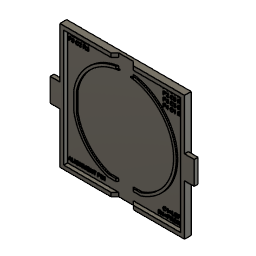
pin_grid_wafer_jig (Autodesk Fusion 360 design; units mm, degrees)
part number: 2026-08-11-19-59-54-396
Autodesk Fusion 360 part; units mm, degrees
ref_plane "WorkPlane1" through (0, 0, 3) normal (0, 0, 1) x (1, 0, 0)
ref_plane "WorkPlane2" through (0, 0, 4.7) normal (0, 0, 1) x (1, 0, 0)
ref_plane "WorkPlane3" through (0, 0, 7.2) normal (0, 0, 1) x (1, 0, 0)
ref_plane "WorkPlane4" through (0, 0, -5) normal (0, 0, 1) x (1, 0, 0)
ref_plane "WorkPlane5" through (0, 0, -4) normal (0, 0, 1) x (1, 0, 0)
sketch "128 mm Square Wafer Platform Sketch" plane through (0, 0, 0) normal (0, 0, 1) x (1, 0, 0)
  line L0 (-53.693, -70.236) -> (74.307, -70.236)
  line L1 (74.307, -70.236) -> (74.307, 57.764)
  line L2 (74.307, 57.764) -> (-53.693, 57.764)
  line L3 (-53.693, 57.764) -> (-53.693, -70.236)
extrude "128 mm Square Wafer Platform" add sketch "128 mm Square Wafer Platform Sketch" along normal blind 3
sketch "4 x 4 mm Perimeter Reinforcement Bar Sketch" plane through (0, 0, 3) normal (0, 0, 1) x (1, 0, 0)
  line L0 (-53.693, -70.236) -> (74.307, -70.236)
  line L1 (74.307, -70.236) -> (74.307, 57.764)
  line L2 (74.307, 57.764) -> (-53.693, 57.764)
  line L3 (-53.693, 57.764) -> (-53.693, -70.236)
  line L4 (-49.693, -66.236) -> (70.307, -66.236)
  line L5 (70.307, -66.236) -> (70.307, 53.764)
  line L6 (70.307, 53.764) -> (-49.693, 53.764)
  line L7 (-49.693, 53.764) -> (-49.693, -66.236)
extrude "4 x 4 mm Perimeter Reinforcement Bar" add sketch "4 x 4 mm Perimeter Reinforcement Bar Sketch" along normal blind 4
sketch "Left Pickup Tab Sketch" plane through (0, 0, 3) normal (0, 0, 1) x (1, 0, 0)
  line L0 (-63.693, -18.236) -> (-53.693, -18.236)
  line L1 (-53.693, -18.236) -> (-53.693, 5.764)
  line L2 (-53.693, 5.764) -> (-63.693, 5.764)
  line L3 (-63.693, 5.764) -> (-63.693, -18.236)
extrude "Left Pickup Tab" add sketch "Left Pickup Tab Sketch" along normal blind 4
sketch "Right Pickup Tab Sketch" plane through (0, 0, 3) normal (0, 0, 1) x (1, 0, 0)
  line L0 (74.307, -18.236) -> (84.307, -18.236)
  line L1 (84.307, -18.236) -> (84.307, 5.764)
  line L2 (84.307, 5.764) -> (74.307, 5.764)
  line L3 (74.307, 5.764) -> (74.307, -18.236)
extrude "Right Pickup Tab" add sketch "Right Pickup Tab Sketch" along normal blind 4
sketch "15 mm Outer Bar Tweezer Notch with 45 Degree Sides Lower Sketch" plane through (0, 0, 3) normal (0, 0, 1) x (1, 0, 0)
  line L0 (2.807, -70.336) -> (17.807, -70.336)
  line L1 (17.807, -70.336) -> (17.807, -66.136)
  line L2 (17.807, -66.136) -> (2.807, -66.136)
  line L3 (2.807, -66.136) -> (2.807, -70.336)
sketch "15 mm Outer Bar Tweezer Notch with 45 Degree Sides Upper Sketch" plane through (0, 0, 7.2) normal (0, 0, 1) x (1, 0, 0)
  line L0 (-1.393, -74.536) -> (22.007, -74.536)
  line L1 (22.007, -74.536) -> (22.007, -61.936)
  line L2 (22.007, -61.936) -> (-1.393, -61.936)
  line L3 (-1.393, -61.936) -> (-1.393, -74.536)
loft "15 mm Outer Bar Tweezer Notch with 45 Degree Sides" cut profiles "15 mm Outer Bar Tweezer Notch with 45 Degree Sides Lower Sketch", "15 mm Outer Bar Tweezer Notch with 45 Degree Sides Upper Sketch" section 1 section 2
sketch "1.5 mm Raised Wafer Nest Sketch" plane through (0, 0, 3) normal (0, 0, 1) x (1, 0, 0)
  line L0 (63.307, -6.236) -> (63.2747, -4.3863)
  line L1 (63.2747, -4.3863) -> (63.1779, -2.5389)
  line L2 (63.1779, -2.5389) -> (63.0167, -0.696)
  line L3 (63.0167, -0.696) -> (62.7912, 1.1402)
  line L4 (62.7912, 1.1402) -> (62.5018, 2.9674)
  line L5 (62.5018, 2.9674) -> (62.1488, 4.7833)
  line L6 (62.1488, 4.7833) -> (61.7327, 6.5859)
  line L7 (61.7327, 6.5859) -> (61.2539, 8.3728)
  line L8 (61.2539, 8.3728) -> (60.713, 10.1419)
  line L9 (60.713, 10.1419) -> (60.1107, 11.8911)
  line L10 (60.1107, 11.8911) -> (59.4477, 13.6181)
  line L11 (59.4477, 13.6181) -> (58.7249, 15.321)
  line L12 (58.7249, 15.321) -> (57.9431, 16.9977)
  line L13 (57.9431, 16.9977) -> (57.1032, 18.646)
  line L14 (57.1032, 18.646) -> (56.2063, 20.264)
  line L15 (56.2063, 20.264) -> (55.2535, 21.8497)
  line L16 (55.2535, 21.8497) -> (54.246, 23.4012)
  line L17 (54.246, 23.4012) -> (53.1849, 24.9166)
  line L18 (53.1849, 24.9166) -> (52.0716, 26.3941)
  line L19 (52.0716, 26.3941) -> (50.9074, 27.8317)
  line L20 (50.9074, 27.8317) -> (49.6937, 29.2279)
  line L21 (49.6937, 29.2279) -> (48.432, 30.5809)
  line L22 (48.432, 30.5809) -> (47.1239, 31.889)
  line L23 (47.1239, 31.889) -> (45.7709, 33.1507)
  line L24 (45.7709, 33.1507) -> (44.3747, 34.3644)
  line L25 (44.3747, 34.3644) -> (42.9371, 35.5286)
  line L26 (42.9371, 35.5286) -> (41.4596, 36.6419)
  line L27 (41.4596, 36.6419) -> (39.9442, 37.703)
  line L28 (39.9442, 37.703) -> (38.3927, 38.7105)
  line L29 (38.3927, 38.7105) -> (36.807, 39.6633)
  line L30 (36.807, 39.6633) -> (35.189, 40.5602)
  line L31 (35.189, 40.5602) -> (33.5407, 41.4001)
  line L32 (33.5407, 41.4001) -> (31.864, 42.1819)
  line L33 (31.864, 42.1819) -> (30.1611, 42.9047)
  line L34 (30.1611, 42.9047) -> (28.4341, 43.5677)
  line L35 (28.4341, 43.5677) -> (26.6849, 44.17)
  line L36 (26.6849, 44.17) -> (24.9158, 44.7109)
  line L37 (24.9158, 44.7109) -> (23.1289, 45.1897)
  line L38 (23.1289, 45.1897) -> (21.3263, 45.6058)
  line L39 (21.3263, 45.6058) -> (19.5104, 45.9588)
  line L40 (19.5104, 45.9588) -> (17.6832, 46.2482)
  line L41 (17.6832, 46.2482) -> (15.847, 46.4737)
  line L42 (15.847, 46.4737) -> (14.0041, 46.6349)
  line L43 (14.0041, 46.6349) -> (12.1567, 46.7317)
  line L44 (12.1567, 46.7317) -> (10.307, 46.764)
  line L45 (10.307, 46.764) -> (8.4573, 46.7317)
  line L46 (8.4573, 46.7317) -> (6.6099, 46.6349)
  line L47 (6.6099, 46.6349) -> (4.767, 46.4737)
  line L48 (4.767, 46.4737) -> (2.9308, 46.2482)
  line L49 (2.9308, 46.2482) -> (1.1036, 45.9588)
  line L50 (1.1036, 45.9588) -> (-0.7123, 45.6058)
  line L51 (-0.7123, 45.6058) -> (-2.5149, 45.1897)
  line L52 (-2.5149, 45.1897) -> (-4.3018, 44.7109)
  line L53 (-4.3018, 44.7109) -> (-6.0709, 44.17)
  line L54 (-6.0709, 44.17) -> (-7.8201, 43.5677)
  line L55 (-7.8201, 43.5677) -> (-9.5471, 42.9047)
  line L56 (-9.5471, 42.9047) -> (-11.25, 42.1819)
  line L57 (-11.25, 42.1819) -> (-12.9267, 41.4001)
  line L58 (-12.9267, 41.4001) -> (-14.575, 40.5602)
  line L59 (-14.575, 40.5602) -> (-16.193, 39.6633)
  line L60 (-16.193, 39.6633) -> (-17.7787, 38.7105)
  line L61 (-17.7787, 38.7105) -> (-19.3302, 37.703)
  line L62 (-19.3302, 37.703) -> (-20.8456, 36.6419)
  line L63 (-20.8456, 36.6419) -> (-22.3231, 35.5286)
  line L64 (-22.3231, 35.5286) -> (-23.7607, 34.3644)
  line L65 (-23.7607, 34.3644) -> (-25.1569, 33.1507)
  line L66 (-25.1569, 33.1507) -> (-26.5099, 31.889)
  line L67 (-26.5099, 31.889) -> (-27.818, 30.5809)
  line L68 (-27.818, 30.5809) -> (-29.0797, 29.2279)
  line L69 (-29.0797, 29.2279) -> (-30.2934, 27.8317)
  line L70 (-30.2934, 27.8317) -> (-31.4576, 26.3941)
  line L71 (-31.4576, 26.3941) -> (-32.5709, 24.9166)
  line L72 (-32.5709, 24.9166) -> (-33.632, 23.4012)
  line L73 (-33.632, 23.4012) -> (-34.6395, 21.8497)
  line L74 (-34.6395, 21.8497) -> (-35.5923, 20.264)
  line L75 (-35.5923, 20.264) -> (-36.4892, 18.646)
  line L76 (-36.4892, 18.646) -> (-37.3291, 16.9977)
  line L77 (-37.3291, 16.9977) -> (-38.1109, 15.321)
  line L78 (-38.1109, 15.321) -> (-38.8337, 13.6181)
  line L79 (-38.8337, 13.6181) -> (-39.4967, 11.8911)
  line L80 (-39.4967, 11.8911) -> (-40.099, 10.1419)
  line L81 (-40.099, 10.1419) -> (-40.6399, 8.3728)
  line L82 (-40.6399, 8.3728) -> (-41.1187, 6.5859)
  line L83 (-41.1187, 6.5859) -> (-41.5348, 4.7833)
  line L84 (-41.5348, 4.7833) -> (-41.8763, 3.0264)
  line L85 (-41.8763, 3.0264) -> (-41.8763, -15.4984)
  line L86 (-41.8763, -15.4984) -> (-41.5348, -17.2553)
  line L87 (-41.5348, -17.2553) -> (-41.1187, -19.0579)
  line L88 (-41.1187, -19.0579) -> (-40.6399, -20.8448)
  line L89 (-40.6399, -20.8448) -> (-40.099, -22.6139)
  line L90 (-40.099, -22.6139) -> (-39.4967, -24.3631)
  line L91 (-39.4967, -24.3631) -> (-38.8337, -26.0901)
  line L92 (-38.8337, -26.0901) -> (-38.1109, -27.793)
  line L93 (-38.1109, -27.793) -> (-37.3291, -29.4697)
  line L94 (-37.3291, -29.4697) -> (-36.4892, -31.118)
  line L95 (-36.4892, -31.118) -> (-35.5923, -32.736)
  line L96 (-35.5923, -32.736) -> (-34.6395, -34.3217)
  line L97 (-34.6395, -34.3217) -> (-33.632, -35.8732)
  line L98 (-33.632, -35.8732) -> (-32.5709, -37.3886)
  line L99 (-32.5709, -37.3886) -> (-31.4576, -38.8661)
  line L100 (-31.4576, -38.8661) -> (-30.2934, -40.3037)
  line L101 (-30.2934, -40.3037) -> (-29.0797, -41.6999)
  line L102 (-29.0797, -41.6999) -> (-27.818, -43.0529)
  line L103 (-27.818, -43.0529) -> (-26.5099, -44.361)
  line L104 (-26.5099, -44.361) -> (-25.1569, -45.6227)
  line L105 (-25.1569, -45.6227) -> (-23.7607, -46.8364)
  line L106 (-23.7607, -46.8364) -> (-22.3231, -48.0006)
  line L107 (-22.3231, -48.0006) -> (-20.8456, -49.1139)
  line L108 (-20.8456, -49.1139) -> (-19.3302, -50.175)
  line L109 (-19.3302, -50.175) -> (-17.7787, -51.1825)
  line L110 (-17.7787, -51.1825) -> (-16.193, -52.1353)
  line L111 (-16.193, -52.1353) -> (-14.575, -53.0322)
  line L112 (-14.575, -53.0322) -> (-12.9267, -53.8721)
  line L113 (-12.9267, -53.8721) -> (-11.25, -54.6539)
  line L114 (-11.25, -54.6539) -> (-9.5471, -55.3767)
  line L115 (-9.5471, -55.3767) -> (-7.8201, -56.0397)
  line L116 (-7.8201, -56.0397) -> (-6.4203, -56.5217)
  line L117 (-6.4203, -56.5217) -> (27.0343, -56.5217)
  line L118 (27.0343, -56.5217) -> (28.4341, -56.0397)
  line L119 (28.4341, -56.0397) -> (30.1611, -55.3767)
  line L120 (30.1611, -55.3767) -> (31.864, -54.6539)
  line L121 (31.864, -54.6539) -> (33.5407, -53.8721)
  line L122 (33.5407, -53.8721) -> (35.189, -53.0322)
  line L123 (35.189, -53.0322) -> (36.807, -52.1353)
  line L124 (36.807, -52.1353) -> (38.3927, -51.1825)
  line L125 (38.3927, -51.1825) -> (39.9442, -50.175)
  line L126 (39.9442, -50.175) -> (41.4596, -49.1139)
  line L127 (41.4596, -49.1139) -> (42.9371, -48.0006)
  line L128 (42.9371, -48.0006) -> (44.3747, -46.8364)
  line L129 (44.3747, -46.8364) -> (45.7709, -45.6227)
  line L130 (45.7709, -45.6227) -> (47.1239, -44.361)
  line L131 (47.1239, -44.361) -> (48.432, -43.0529)
  line L132 (48.432, -43.0529) -> (49.6937, -41.6999)
  line L133 (49.6937, -41.6999) -> (50.9074, -40.3037)
  line L134 (50.9074, -40.3037) -> (52.0716, -38.8661)
  line L135 (52.0716, -38.8661) -> (53.1849, -37.3886)
  line L136 (53.1849, -37.3886) -> (54.246, -35.8732)
  line L137 (54.246, -35.8732) -> (55.2535, -34.3217)
  line L138 (55.2535, -34.3217) -> (56.2063, -32.736)
  line L139 (56.2063, -32.736) -> (57.1032, -31.118)
  line L140 (57.1032, -31.118) -> (57.9431, -29.4697)
  line L141 (57.9431, -29.4697) -> (58.7249, -27.793)
  line L142 (58.7249, -27.793) -> (59.4477, -26.0901)
  line L143 (59.4477, -26.0901) -> (60.1107, -24.3631)
  line L144 (60.1107, -24.3631) -> (60.713, -22.6139)
  line L145 (60.713, -22.6139) -> (61.2539, -20.8448)
  line L146 (61.2539, -20.8448) -> (61.7327, -19.0579)
  line L147 (61.7327, -19.0579) -> (62.1488, -17.2553)
  line L148 (62.1488, -17.2553) -> (62.5018, -15.4394)
  line L149 (62.5018, -15.4394) -> (62.7912, -13.6122)
  line L150 (62.7912, -13.6122) -> (63.0167, -11.776)
  line L151 (63.0167, -11.776) -> (63.1779, -9.9331)
  line L152 (63.1779, -9.9331) -> (63.2747, -8.0857)
  line L153 (63.2747, -8.0857) -> (63.307, -6.236)
extrude "1.5 mm Raised Wafer Nest" add sketch "1.5 mm Raised Wafer Nest Sketch" along normal blind 1.5
sketch "Final Wafer Pocket Clearance Sketch" plane through (0, 0, 3) normal (0, 0, 1) x (1, 0, 0)
  line L0 (60.632, -6.236) -> (60.6013, -4.4797)
  line L1 (60.6013, -4.4797) -> (60.5094, -2.7255)
  line L2 (60.5094, -2.7255) -> (60.3563, -0.9756)
  line L3 (60.3563, -0.9756) -> (60.1422, 0.7679)
  line L4 (60.1422, 0.7679) -> (59.8675, 2.5028)
  line L5 (59.8675, 2.5028) -> (59.5323, 4.2272)
  line L6 (59.5323, 4.2272) -> (59.1371, 5.9387)
  line L7 (59.1371, 5.9387) -> (58.6825, 7.6354)
  line L8 (58.6825, 7.6354) -> (58.1689, 9.3153)
  line L9 (58.1689, 9.3153) -> (57.597, 10.9762)
  line L10 (57.597, 10.9762) -> (56.9675, 12.6161)
  line L11 (56.9675, 12.6161) -> (56.2812, 14.233)
  line L12 (56.2812, 14.233) -> (55.5388, 15.825)
  line L13 (55.5388, 15.825) -> (54.7413, 17.3902)
  line L14 (54.7413, 17.3902) -> (53.8897, 18.9265)
  line L15 (53.8897, 18.9265) -> (52.985, 20.4322)
  line L16 (52.985, 20.4322) -> (52.0283, 21.9054)
  line L17 (52.0283, 21.9054) -> (51.0208, 23.3443)
  line L18 (51.0208, 23.3443) -> (49.9636, 24.7472)
  line L19 (49.9636, 24.7472) -> (48.8582, 26.1123)
  line L20 (48.8582, 26.1123) -> (47.7058, 27.438)
  line L21 (47.7058, 27.438) -> (46.5078, 28.7227)
  line L22 (46.5078, 28.7227) -> (45.2657, 29.9648)
  line L23 (45.2657, 29.9648) -> (43.981, 31.1628)
  line L24 (43.981, 31.1628) -> (42.6553, 32.3152)
  line L25 (42.6553, 32.3152) -> (41.2902, 33.4206)
  line L26 (41.2902, 33.4206) -> (39.8873, 34.4778)
  line L27 (39.8873, 34.4778) -> (38.4484, 35.4853)
  line L28 (38.4484, 35.4853) -> (36.9752, 36.442)
  line L29 (36.9752, 36.442) -> (35.4695, 37.3467)
  line L30 (35.4695, 37.3467) -> (33.9332, 38.1983)
  line L31 (33.9332, 38.1983) -> (32.368, 38.9958)
  line L32 (32.368, 38.9958) -> (30.776, 39.7382)
  line L33 (30.776, 39.7382) -> (29.1591, 40.4245)
  line L34 (29.1591, 40.4245) -> (27.5192, 41.054)
  line L35 (27.5192, 41.054) -> (25.8583, 41.6259)
  line L36 (25.8583, 41.6259) -> (24.1784, 42.1395)
  line L37 (24.1784, 42.1395) -> (22.4817, 42.5941)
  line L38 (22.4817, 42.5941) -> (20.7702, 42.9893)
  line L39 (20.7702, 42.9893) -> (19.0458, 43.3245)
  line L40 (19.0458, 43.3245) -> (17.3109, 43.5992)
  line L41 (17.3109, 43.5992) -> (15.5674, 43.8133)
  line L42 (15.5674, 43.8133) -> (13.8175, 43.9664)
  line L43 (13.8175, 43.9664) -> (12.0633, 44.0583)
  line L44 (12.0633, 44.0583) -> (10.307, 44.089)
  line L45 (10.307, 44.089) -> (8.5507, 44.0583)
  line L46 (8.5507, 44.0583) -> (6.7965, 43.9664)
  line L47 (6.7965, 43.9664) -> (5.0466, 43.8133)
  line L48 (5.0466, 43.8133) -> (3.3031, 43.5992)
  line L49 (3.3031, 43.5992) -> (1.5682, 43.3245)
  line L50 (1.5682, 43.3245) -> (-0.1562, 42.9893)
  line L51 (-0.1562, 42.9893) -> (-1.8677, 42.5941)
  line L52 (-1.8677, 42.5941) -> (-3.5644, 42.1395)
  line L53 (-3.5644, 42.1395) -> (-5.2443, 41.6259)
  line L54 (-5.2443, 41.6259) -> (-6.9052, 41.054)
  line L55 (-6.9052, 41.054) -> (-8.5451, 40.4245)
  line L56 (-8.5451, 40.4245) -> (-10.162, 39.7382)
  line L57 (-10.162, 39.7382) -> (-11.754, 38.9958)
  line L58 (-11.754, 38.9958) -> (-13.3192, 38.1983)
  line L59 (-13.3192, 38.1983) -> (-14.8555, 37.3467)
  line L60 (-14.8555, 37.3467) -> (-16.3612, 36.442)
  line L61 (-16.3612, 36.442) -> (-17.8344, 35.4853)
  line L62 (-17.8344, 35.4853) -> (-19.2733, 34.4778)
  line L63 (-19.2733, 34.4778) -> (-20.6762, 33.4206)
  line L64 (-20.6762, 33.4206) -> (-22.0413, 32.3152)
  line L65 (-22.0413, 32.3152) -> (-23.367, 31.1628)
  line L66 (-23.367, 31.1628) -> (-24.6517, 29.9648)
  line L67 (-24.6517, 29.9648) -> (-25.8938, 28.7227)
  line L68 (-25.8938, 28.7227) -> (-27.0918, 27.438)
  line L69 (-27.0918, 27.438) -> (-28.2442, 26.1123)
  line L70 (-28.2442, 26.1123) -> (-29.3496, 24.7472)
  line L71 (-29.3496, 24.7472) -> (-30.4068, 23.3443)
  line L72 (-30.4068, 23.3443) -> (-31.4143, 21.9054)
  line L73 (-31.4143, 21.9054) -> (-32.371, 20.4322)
  line L74 (-32.371, 20.4322) -> (-33.2757, 18.9265)
  line L75 (-33.2757, 18.9265) -> (-34.1273, 17.3902)
  line L76 (-34.1273, 17.3902) -> (-34.9248, 15.825)
  line L77 (-34.9248, 15.825) -> (-35.6672, 14.233)
  line L78 (-35.6672, 14.233) -> (-36.3535, 12.6161)
  line L79 (-36.3535, 12.6161) -> (-36.983, 10.9762)
  line L80 (-36.983, 10.9762) -> (-37.5549, 9.3153)
  line L81 (-37.5549, 9.3153) -> (-38.0685, 7.6354)
  line L82 (-38.0685, 7.6354) -> (-38.5231, 5.9387)
  line L83 (-38.5231, 5.9387) -> (-38.9183, 4.2272)
  line L84 (-38.9183, 4.2272) -> (-39.0713, 3.4398)
  line L85 (-39.0713, 3.4398) -> (-39.0713, -15.9118)
  line L86 (-39.0713, -15.9118) -> (-38.9183, -16.6992)
  line L87 (-38.9183, -16.6992) -> (-38.5231, -18.4107)
  line L88 (-38.5231, -18.4107) -> (-38.0685, -20.1074)
  line L89 (-38.0685, -20.1074) -> (-37.5549, -21.7873)
  line L90 (-37.5549, -21.7873) -> (-36.983, -23.4482)
  line L91 (-36.983, -23.4482) -> (-36.3535, -25.0881)
  line L92 (-36.3535, -25.0881) -> (-35.6672, -26.705)
  line L93 (-35.6672, -26.705) -> (-34.9248, -28.297)
  line L94 (-34.9248, -28.297) -> (-34.1273, -29.8622)
  line L95 (-34.1273, -29.8622) -> (-33.2757, -31.3985)
  line L96 (-33.2757, -31.3985) -> (-32.371, -32.9042)
  line L97 (-32.371, -32.9042) -> (-31.4143, -34.3774)
  line L98 (-31.4143, -34.3774) -> (-30.4068, -35.8163)
  line L99 (-30.4068, -35.8163) -> (-29.3496, -37.2192)
  line L100 (-29.3496, -37.2192) -> (-28.2442, -38.5843)
  line L101 (-28.2442, -38.5843) -> (-27.0918, -39.91)
  line L102 (-27.0918, -39.91) -> (-25.8938, -41.1947)
  line L103 (-25.8938, -41.1947) -> (-24.6517, -42.4368)
  line L104 (-24.6517, -42.4368) -> (-23.367, -43.6348)
  line L105 (-23.367, -43.6348) -> (-22.0413, -44.7872)
  line L106 (-22.0413, -44.7872) -> (-20.6762, -45.8926)
  line L107 (-20.6762, -45.8926) -> (-19.2733, -46.9498)
  line L108 (-19.2733, -46.9498) -> (-17.8344, -47.9573)
  line L109 (-17.8344, -47.9573) -> (-16.3612, -48.914)
  line L110 (-16.3612, -48.914) -> (-14.8555, -49.8187)
  line L111 (-14.8555, -49.8187) -> (-13.3192, -50.6703)
  line L112 (-13.3192, -50.6703) -> (-11.754, -51.4678)
  line L113 (-11.754, -51.4678) -> (-10.162, -52.2102)
  line L114 (-10.162, -52.2102) -> (-8.5451, -52.8965)
  line L115 (-8.5451, -52.8965) -> (-6.9052, -53.526)
  line L116 (-6.9052, -53.526) -> (-5.9739, -53.8467)
  line L117 (-5.9739, -53.8467) -> (26.5879, -53.8467)
  line L118 (26.5879, -53.8467) -> (27.5192, -53.526)
  line L119 (27.5192, -53.526) -> (29.1591, -52.8965)
  line L120 (29.1591, -52.8965) -> (30.776, -52.2102)
  line L121 (30.776, -52.2102) -> (32.368, -51.4678)
  line L122 (32.368, -51.4678) -> (33.9332, -50.6703)
  line L123 (33.9332, -50.6703) -> (35.4695, -49.8187)
  line L124 (35.4695, -49.8187) -> (36.9752, -48.914)
  line L125 (36.9752, -48.914) -> (38.4484, -47.9573)
  line L126 (38.4484, -47.9573) -> (39.8873, -46.9498)
  line L127 (39.8873, -46.9498) -> (41.2902, -45.8926)
  line L128 (41.2902, -45.8926) -> (42.6553, -44.7872)
  line L129 (42.6553, -44.7872) -> (43.981, -43.6348)
  line L130 (43.981, -43.6348) -> (45.2657, -42.4368)
  line L131 (45.2657, -42.4368) -> (46.5078, -41.1947)
  line L132 (46.5078, -41.1947) -> (47.7058, -39.91)
  line L133 (47.7058, -39.91) -> (48.8582, -38.5843)
  line L134 (48.8582, -38.5843) -> (49.9636, -37.2192)
  line L135 (49.9636, -37.2192) -> (51.0208, -35.8163)
  line L136 (51.0208, -35.8163) -> (52.0283, -34.3774)
  line L137 (52.0283, -34.3774) -> (52.985, -32.9042)
  line L138 (52.985, -32.9042) -> (53.8897, -31.3985)
  line L139 (53.8897, -31.3985) -> (54.7413, -29.8622)
  line L140 (54.7413, -29.8622) -> (55.5388, -28.297)
  line L141 (55.5388, -28.297) -> (56.2812, -26.705)
  line L142 (56.2812, -26.705) -> (56.9675, -25.0881)
  line L143 (56.9675, -25.0881) -> (57.597, -23.4482)
  line L144 (57.597, -23.4482) -> (58.1689, -21.7873)
  line L145 (58.1689, -21.7873) -> (58.6825, -20.1074)
  line L146 (58.6825, -20.1074) -> (59.1371, -18.4107)
  line L147 (59.1371, -18.4107) -> (59.5323, -16.6992)
  line L148 (59.5323, -16.6992) -> (59.8675, -14.9748)
  line L149 (59.8675, -14.9748) -> (60.1422, -13.2399)
  line L150 (60.1422, -13.2399) -> (60.3563, -11.4964)
  line L151 (60.3563, -11.4964) -> (60.5094, -9.7465)
  line L152 (60.5094, -9.7465) -> (60.6013, -7.9923)
  line L153 (60.6013, -7.9923) -> (60.632, -6.236)
extrude "Final Wafer Pocket Clearance" cut sketch "Final Wafer Pocket Clearance Sketch" along normal blind 1.6
sketch "15 mm Pickup Opening with 45 Degree Bevel Lower Sketch" plane through (0, 0, 3) normal (0, 0, 1) x (1, 0, 0)
  line L0 (2.807, -56.5217) -> (2.807, -53.5217)
  line L1 (2.807, -53.5217) -> (2.8542, -52.682)
  line L2 (2.8542, -52.682) -> (2.995, -51.8528)
  line L3 (2.995, -51.8528) -> (3.2279, -51.0446)
  line L4 (3.2279, -51.0446) -> (3.5497, -50.2676)
  line L5 (3.5497, -50.2676) -> (3.9566, -49.5315)
  line L6 (3.9566, -49.5315) -> (4.4433, -48.8455)
  line L7 (4.4433, -48.8455) -> (5.0037, -48.2184)
  line L8 (5.0037, -48.2184) -> (5.6308, -47.658)
  line L9 (5.6308, -47.658) -> (6.3168, -47.1713)
  line L10 (6.3168, -47.1713) -> (7.0529, -46.7644)
  line L11 (7.0529, -46.7644) -> (7.8299, -46.4426)
  line L12 (7.8299, -46.4426) -> (8.6381, -46.2097)
  line L13 (8.6381, -46.2097) -> (9.4673, -46.0689)
  line L14 (9.4673, -46.0689) -> (10.307, -46.0217)
  line L15 (10.307, -46.0217) -> (11.1467, -46.0689)
  line L16 (11.1467, -46.0689) -> (11.9759, -46.2097)
  line L17 (11.9759, -46.2097) -> (12.7841, -46.4426)
  line L18 (12.7841, -46.4426) -> (13.5611, -46.7644)
  line L19 (13.5611, -46.7644) -> (14.2972, -47.1713)
  line L20 (14.2972, -47.1713) -> (14.9832, -47.658)
  line L21 (14.9832, -47.658) -> (15.6103, -48.2184)
  line L22 (15.6103, -48.2184) -> (16.1707, -48.8455)
  line L23 (16.1707, -48.8455) -> (16.6574, -49.5315)
  line L24 (16.6574, -49.5315) -> (17.0643, -50.2676)
  line L25 (17.0643, -50.2676) -> (17.3861, -51.0446)
  line L26 (17.3861, -51.0446) -> (17.619, -51.8528)
  line L27 (17.619, -51.8528) -> (17.7598, -52.682)
  line L28 (17.7598, -52.682) -> (17.807, -53.5217)
  line L29 (17.807, -53.5217) -> (17.807, -56.5217)
  line L30 (17.807, -56.5217) -> (17.7598, -57.3614)
  line L31 (17.7598, -57.3614) -> (17.619, -58.1906)
  line L32 (17.619, -58.1906) -> (17.3861, -58.9988)
  line L33 (17.3861, -58.9988) -> (17.0643, -59.7758)
  line L34 (17.0643, -59.7758) -> (16.6574, -60.5119)
  line L35 (16.6574, -60.5119) -> (16.1707, -61.1979)
  line L36 (16.1707, -61.1979) -> (15.6103, -61.825)
  line L37 (15.6103, -61.825) -> (14.9832, -62.3854)
  line L38 (14.9832, -62.3854) -> (14.2972, -62.8721)
  line L39 (14.2972, -62.8721) -> (13.5611, -63.279)
  line L40 (13.5611, -63.279) -> (12.7841, -63.6008)
  line L41 (12.7841, -63.6008) -> (11.9759, -63.8337)
  line L42 (11.9759, -63.8337) -> (11.1467, -63.9745)
  line L43 (11.1467, -63.9745) -> (10.307, -64.0217)
  line L44 (10.307, -64.0217) -> (9.4673, -63.9745)
  line L45 (9.4673, -63.9745) -> (8.6381, -63.8337)
  line L46 (8.6381, -63.8337) -> (7.8299, -63.6008)
  line L47 (7.8299, -63.6008) -> (7.0529, -63.279)
  line L48 (7.0529, -63.279) -> (6.3168, -62.8721)
  line L49 (6.3168, -62.8721) -> (5.6308, -62.3854)
  line L50 (5.6308, -62.3854) -> (5.0037, -61.825)
  line L51 (5.0037, -61.825) -> (4.4433, -61.1979)
  line L52 (4.4433, -61.1979) -> (3.9566, -60.5119)
  line L53 (3.9566, -60.5119) -> (3.5497, -59.7758)
  line L54 (3.5497, -59.7758) -> (3.2279, -58.9988)
  line L55 (3.2279, -58.9988) -> (2.995, -58.1906)
  line L56 (2.995, -58.1906) -> (2.8542, -57.3614)
  line L57 (2.8542, -57.3614) -> (2.807, -56.5217)
sketch "15 mm Pickup Opening with 45 Degree Bevel Upper Sketch" plane through (0, 0, 4.7) normal (0, 0, 1) x (1, 0, 0)
  line L0 (1.107, -58.2217) -> (1.107, -51.8217)
  line L1 (1.107, -51.8217) -> (1.1648, -50.7916)
  line L2 (1.1648, -50.7916) -> (1.3377, -49.7745)
  line L3 (1.3377, -49.7745) -> (1.6233, -48.7831)
  line L4 (1.6233, -48.7831) -> (2.0181, -47.83)
  line L5 (2.0181, -47.83) -> (2.5171, -46.927)
  line L6 (2.5171, -46.927) -> (3.1142, -46.0856)
  line L7 (3.1142, -46.0856) -> (3.8016, -45.3163)
  line L8 (3.8016, -45.3163) -> (4.5709, -44.6289)
  line L9 (4.5709, -44.6289) -> (5.4123, -44.0318)
  line L10 (5.4123, -44.0318) -> (6.3153, -43.5328)
  line L11 (6.3153, -43.5328) -> (7.2684, -43.138)
  line L12 (7.2684, -43.138) -> (8.2598, -42.8524)
  line L13 (8.2598, -42.8524) -> (9.2769, -42.6795)
  line L14 (9.2769, -42.6795) -> (10.307, -42.6217)
  line L15 (10.307, -42.6217) -> (11.3371, -42.6795)
  line L16 (11.3371, -42.6795) -> (12.3542, -42.8524)
  line L17 (12.3542, -42.8524) -> (13.3456, -43.138)
  line L18 (13.3456, -43.138) -> (14.2987, -43.5328)
  line L19 (14.2987, -43.5328) -> (15.2017, -44.0318)
  line L20 (15.2017, -44.0318) -> (16.0431, -44.6289)
  line L21 (16.0431, -44.6289) -> (16.8124, -45.3163)
  line L22 (16.8124, -45.3163) -> (17.4998, -46.0856)
  line L23 (17.4998, -46.0856) -> (18.0969, -46.927)
  line L24 (18.0969, -46.927) -> (18.5959, -47.83)
  line L25 (18.5959, -47.83) -> (18.9907, -48.7831)
  line L26 (18.9907, -48.7831) -> (19.2763, -49.7745)
  line L27 (19.2763, -49.7745) -> (19.4492, -50.7916)
  line L28 (19.4492, -50.7916) -> (19.507, -51.8217)
  line L29 (19.507, -51.8217) -> (19.507, -58.2217)
  line L30 (19.507, -58.2217) -> (19.4492, -59.2518)
  line L31 (19.4492, -59.2518) -> (19.2763, -60.2689)
  line L32 (19.2763, -60.2689) -> (18.9907, -61.2603)
  line L33 (18.9907, -61.2603) -> (18.5959, -62.2134)
  line L34 (18.5959, -62.2134) -> (18.0969, -63.1164)
  line L35 (18.0969, -63.1164) -> (17.4998, -63.9578)
  line L36 (17.4998, -63.9578) -> (16.8124, -64.7271)
  line L37 (16.8124, -64.7271) -> (16.0431, -65.4146)
  line L38 (16.0431, -65.4146) -> (15.2017, -66.0116)
  line L39 (15.2017, -66.0116) -> (14.2987, -66.5106)
  line L40 (14.2987, -66.5106) -> (13.3456, -66.9054)
  line L41 (13.3456, -66.9054) -> (12.3542, -67.191)
  line L42 (12.3542, -67.191) -> (11.3371, -67.3639)
  line L43 (11.3371, -67.3639) -> (10.307, -67.4217)
  line L44 (10.307, -67.4217) -> (9.2769, -67.3639)
  line L45 (9.2769, -67.3639) -> (8.2598, -67.191)
  line L46 (8.2598, -67.191) -> (7.2684, -66.9054)
  line L47 (7.2684, -66.9054) -> (6.3153, -66.5106)
  line L48 (6.3153, -66.5106) -> (5.4123, -66.0116)
  line L49 (5.4123, -66.0116) -> (4.5709, -65.4146)
  line L50 (4.5709, -65.4146) -> (3.8016, -64.7271)
  line L51 (3.8016, -64.7271) -> (3.1142, -63.9578)
  line L52 (3.1142, -63.9578) -> (2.5171, -63.1164)
  line L53 (2.5171, -63.1164) -> (2.0181, -62.2134)
  line L54 (2.0181, -62.2134) -> (1.6233, -61.2603)
  line L55 (1.6233, -61.2603) -> (1.3377, -60.2689)
  line L56 (1.3377, -60.2689) -> (1.1648, -59.2518)
  line L57 (1.1648, -59.2518) -> (1.107, -58.2217)
loft "15 mm Pickup Opening with 45 Degree Bevel" cut profiles "15 mm Pickup Opening with 45 Degree Bevel Lower Sketch", "15 mm Pickup Opening with 45 Degree Bevel Upper Sketch" section 1 section 2
sketch "15 mm Rear Tape Gap with 45 Degree Bevel Lower Sketch" plane through (0, 0, 3) normal (0, 0, 1) x (1, 0, 0)
  line L0 (2.807, 43.764) -> (17.807, 43.764)
  line L1 (17.807, 43.764) -> (17.807, 46.964)
  line L2 (17.807, 46.964) -> (2.807, 46.964)
  line L3 (2.807, 46.964) -> (2.807, 43.764)
sketch "15 mm Rear Tape Gap with 45 Degree Bevel Upper Sketch" plane through (0, 0, 4.7) normal (0, 0, 1) x (1, 0, 0)
  line L0 (1.107, 43.764) -> (19.507, 43.764)
  line L1 (19.507, 43.764) -> (19.507, 46.964)
  line L2 (19.507, 46.964) -> (1.107, 46.964)
  line L3 (1.107, 46.964) -> (1.107, 43.764)
loft "15 mm Rear Tape Gap with 45 Degree Bevel" cut profiles "15 mm Rear Tape Gap with 45 Degree Bevel Lower Sketch", "15 mm Rear Tape Gap with 45 Degree Bevel Upper Sketch" section 1 section 2
sketch "15 mm Rear Outer Bar Notch with 45 Degree Sides Lower Sketch" plane through (0, 0, 3) normal (0, 0, 1) x (1, 0, 0)
  line L0 (2.807, 53.664) -> (17.807, 53.664)
  line L1 (17.807, 53.664) -> (17.807, 57.864)
  line L2 (17.807, 57.864) -> (2.807, 57.864)
  line L3 (2.807, 57.864) -> (2.807, 53.664)
sketch "15 mm Rear Outer Bar Notch with 45 Degree Sides Upper Sketch" plane through (0, 0, 7.2) normal (0, 0, 1) x (1, 0, 0)
  line L0 (-1.393, 49.464) -> (22.007, 49.464)
  line L1 (22.007, 49.464) -> (22.007, 62.064)
  line L2 (22.007, 62.064) -> (-1.393, 62.064)
  line L3 (-1.393, 62.064) -> (-1.393, 49.464)
loft "15 mm Rear Outer Bar Notch with 45 Degree Sides" cut profiles "15 mm Rear Outer Bar Notch with 45 Degree Sides Lower Sketch", "15 mm Rear Outer Bar Notch with 45 Degree Sides Upper Sketch" section 1 section 2
sketch "Outer Front Left Pin Cylinder Sketch" plane through (0, 0, -4) normal (0, 0, 1) x (1, 0, 0)
  circle A0 centre (-50.8, -50.8) radius 2.35
extrude "Outer Front Left 4.65 mm Pin" add sketch "Outer Front Left Pin Cylinder Sketch" along normal blind 7
sketch "Outer Front Left Tapered Tip Tip" plane through (0, 0, -5) normal (0, 0, 1) x (1, 0, 0)
  circle A0 centre (-50.8, -50.8) radius 2.025
sketch "Outer Front Left Tapered Tip Shoulder" plane through (0, 0, -4) normal (0, 0, 1) x (1, 0, 0)
  circle A0 centre (-50.8, -50.8) radius 2.35
loft "Outer Front Left Tapered Tip" add profiles "Outer Front Left Tapered Tip Tip", "Outer Front Left Tapered Tip Shoulder" section 1 section 2
sketch "Outer Front Right Pin Cylinder Sketch" plane through (0, 0, -4) normal (0, 0, 1) x (1, 0, 0)
  circle A0 centre (50.8, -50.8) radius 2.35
extrude "Outer Front Right 4.65 mm Pin" add sketch "Outer Front Right Pin Cylinder Sketch" along normal blind 7
sketch "Outer Front Right Tapered Tip Tip" plane through (0, 0, -5) normal (0, 0, 1) x (1, 0, 0)
  circle A0 centre (50.8, -50.8) radius 2.025
sketch "Outer Front Right Tapered Tip Shoulder" plane through (0, 0, -4) normal (0, 0, 1) x (1, 0, 0)
  circle A0 centre (50.8, -50.8) radius 2.35
loft "Outer Front Right Tapered Tip" add profiles "Outer Front Right Tapered Tip Tip", "Outer Front Right Tapered Tip Shoulder" section 1 section 2
sketch "Outer Rear Left Pin Cylinder Sketch" plane through (0, 0, -4) normal (0, 0, 1) x (1, 0, 0)
  circle A0 centre (-50.8, 50.8) radius 2.35
extrude "Outer Rear Left 4.65 mm Pin" add sketch "Outer Rear Left Pin Cylinder Sketch" along normal blind 7
sketch "Outer Rear Left Tapered Tip Tip" plane through (0, 0, -5) normal (0, 0, 1) x (1, 0, 0)
  circle A0 centre (-50.8, 50.8) radius 2.025
sketch "Outer Rear Left Tapered Tip Shoulder" plane through (0, 0, -4) normal (0, 0, 1) x (1, 0, 0)
  circle A0 centre (-50.8, 50.8) radius 2.35
loft "Outer Rear Left Tapered Tip" add profiles "Outer Rear Left Tapered Tip Tip", "Outer Rear Left Tapered Tip Shoulder" section 1 section 2
sketch "Outer Rear Right Pin Cylinder Sketch" plane through (0, 0, -4) normal (0, 0, 1) x (1, 0, 0)
  circle A0 centre (50.8, 50.8) radius 2.35
extrude "Outer Rear Right 4.65 mm Pin" add sketch "Outer Rear Right Pin Cylinder Sketch" along normal blind 7
sketch "Outer Rear Right Tapered Tip Tip" plane through (0, 0, -5) normal (0, 0, 1) x (1, 0, 0)
  circle A0 centre (50.8, 50.8) radius 2.025
sketch "Outer Rear Right Tapered Tip Shoulder" plane through (0, 0, -4) normal (0, 0, 1) x (1, 0, 0)
  circle A0 centre (50.8, 50.8) radius 2.35
loft "Outer Rear Right Tapered Tip" add profiles "Outer Rear Right Tapered Tip Tip", "Outer Rear Right Tapered Tip Shoulder" section 1 section 2
sketch "Title and P0 - 0.5 mm Engraving Sketch" plane through (0, 0, 3) normal (0, 0, 1) x (1, 0, 0)
  line L0 (-48.693, 38.764) -> (-8.693, 38.764) construction
  line L1 (-8.693, 38.764) -> (-8.693, 52.764) construction
  line L2 (-8.693, 52.764) -> (-48.693, 52.764) construction
  line L3 (-48.693, 52.764) -> (-48.693, 38.764) construction
  dimension "d48" = 3.5
  dimension "d49" = 0
  text T0 "ALIGNER\nP0 C2 R3" font "Arial" height 3.5 align left top in box 40 x 14 at (-48.693, 38.764) x (1, 0) y (0, 1) spacing 1 kerned
extrude "Title and P0 - 0.5 mm Engraving" add sketch "Title and P0 - 0.5 mm Engraving Sketch" along normal blind 0.5 text T0
sketch "Position Map - 0.5 mm Engraving Sketch" plane through (0, 0, 3) normal (0, 0, 1) x (1, 0, 0)
  line L0 (29.307, 28.764) -> (69.307, 28.764) construction
  line L1 (69.307, 28.764) -> (69.307, 52.764) construction
  line L2 (69.307, 52.764) -> (29.307, 52.764) construction
  line L3 (29.307, 52.764) -> (29.307, 28.764) construction
  dimension "d52" = 3.5
  dimension "d53" = 0
  text T0 "P1 C1 R4\nP2 C3 R4\nP3 C3 R2\nP4 C1 R2" font "Arial" height 3.5 align right top in box 40 x 24 at (29.307, 28.764) x (1, 0) y (0, 1) spacing 1 kerned
extrude "Position Map - 0.5 mm Engraving" add sketch "Position Map - 0.5 mm Engraving Sketch" along normal blind 0.5 text T0
sketch "Alignment Pin Label - 0.5 mm Engraving Sketch" plane through (0, 0, 3) normal (0, 0, 1) x (1, 0, 0)
  line L0 (-48.693, -65.236) -> (-6.693, -65.236) construction
  line L1 (-6.693, -65.236) -> (-6.693, -59.236) construction
  line L2 (-6.693, -59.236) -> (-48.693, -59.236) construction
  line L3 (-48.693, -59.236) -> (-48.693, -65.236) construction
  dimension "d56" = 3.5
  text T0 "ALIGNMENT PIN" font "Arial" height 3.5 align left top in box 42 x 6 at (-48.693, -65.236) x (1, 0) y (0, 1) spacing 1 kerned
extrude "Alignment Pin Label - 0.5 mm Engraving" add sketch "Alignment Pin Label - 0.5 mm Engraving Sketch" along normal blind 0.5 text T0
sketch "Grid Orientation Label - 0.5 mm Engraving Sketch" plane through (0, 0, 3) normal (0, 0, 1) x (1, 0, 0)
  line L0 (27.307, -65.236) -> (69.307, -65.236) construction
  line L1 (69.307, -65.236) -> (69.307, -55.236) construction
  line L2 (69.307, -55.236) -> (27.307, -55.236) construction
  line L3 (27.307, -55.236) -> (27.307, -65.236) construction
  dimension "d60" = 3.5
  dimension "d61" = 0
  text T0 "C1=LEFT\nR1=FRONT" font "Arial" height 3.5 align right top in box 42 x 10 at (27.307, -65.236) x (1, 0) y (0, 1) spacing 1 kerned
extrude "Grid Orientation Label - 0.5 mm Engraving" add sketch "Grid Orientation Label - 0.5 mm Engraving Sketch" along normal blind 0.5 text T0
equation "gridPitch = 25.4 mm" comment "Table hole-grid pitch"
equation "indexMove = 50.8 mm" comment "Two-grid-space indexing move"
equation "outerPinPatternSpan = 101.6 mm" comment "Four-space outer pin span"
equation "pinDiameter = 4.7 mm" comment "Printed locating pin diameter"
equation "pinEngagement = 5.0 mm" comment "Pin length below platform"
equation "platformSizeX = 128.0 mm" comment "Compact platform width"
equation "platformSizeY = 128.0 mm" comment "Compact platform depth"
equation "baseThickness = 3.0 mm" comment "Wafer platform thickness"
equation "outerBarWidth = 4.0 mm" comment "Perimeter reinforcement width"
equation "outerBarHeight = 4.0 mm" comment "Perimeter reinforcement height"
equation "sidewallHeight = 1.5 mm" comment "Nest lip height above platform"
equation "nestOffsetX = 7.29 mm" comment "Nest X from pin-square center"
equation "nestOffsetY = -4.95 mm" comment "Nest Y from pin-square center"
equation "pickupGapWidth = 15.0 mm" comment "Primary-flat pickup opening"
equation "rearTapeGapWidth = 15.0 mm" comment "Rear tape-access gap in the lip"
equation "annotationDepth = 0.5 mm" comment "Baseplate text engraving depth"
equation "annotationTextHeight = 3.5 mm" comment "Baseplate text height"
equation "d49 = 'ALIGNER\\nP0 C2 R3'"
equation "d53 = 'P1 C1 R4\\nP2 C3 R4\\nP3 C3 R2\\nP4 C1 R2'"
equation "d57 = 'ALIGNMENT PIN'"
equation "d61 = 'C1=LEFT\\nR1=FRONT'"
